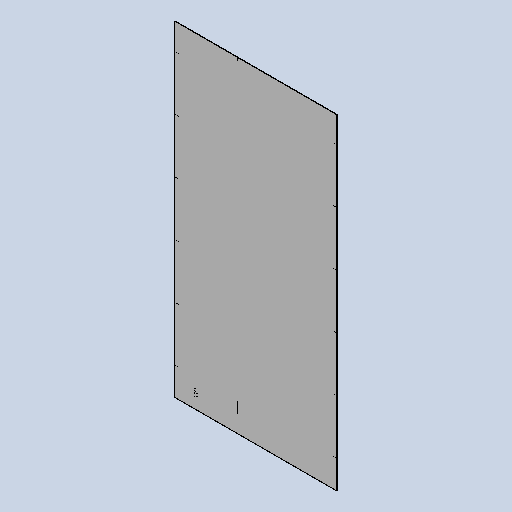
# Autodesk Inventor part: GBK 3122 shield 2
Saved by Autodesk Inventor 2026.2 (Build 302298010, 298A)
## iProperties
Created: 2026-04-17
Part Number: GBK 3122 shield 2
Material: Steel
Document SubType Name: Sheet Metal
Designer: pokla
Stock Number: 3122
Mass: 138487 g
Surface Area: 88564.8 cm^2
Volume: 17641.6 cm^3
Density: 7.85 g/cm^3
Flat Pattern Width: 298 cm
Flat Pattern Length: 148 cm
Flat Pattern Area: 44104 cm^2
Sheet Metal Rule: Default_mm
Sheet Metal Width: 2980,000 мм
Sheet Metal Length: 1480,000 мм
Sheet Metal Area: 4410400,000 мм^2
Appearance: Default
Author: admin
Autodesk Inventor part; units mm, degrees
ref_plane "YZ Plane" through (0, 0, 0) normal (1, 0, 0) x (0, 1, 0)
ref_plane "XZ Plane" through (0, 0, 0) normal (0, 1, 0) x (-1, 0, 0)
ref_plane "XY Plane" through (0, 0, 0) normal (0, 0, 1) x (1, 0, 0)
sketch "Sketch1" plane through (0, 0, 0) normal (0, 0, 1) x (1, 0, 0)
  line L0 (740, -1490) -> (-740, -1490)
  line L1 (-740, -1490) -> (-740, 1490)
  line L2 (-740, 1490) -> (740, 1490)
  line L3 (740, 1490) -> (740, -1490)
  line L4 (740, -1490) -> (-740, 1490) construction
  line L5 (-740, -1490) -> (740, 1490) construction
  point P0 (0, 0)
  dimension "d0" = 1480
  dimension "d1" = 2980
  measures "d0" distance of L1.end L2.end
  measures "d1" distance of L0.end L1.end
extrude "Plate1" add sketch "Sketch1" along normal blind 4
sketch "Эскиз5" plane through (0, 0, 0) normal (0, 0, -1) x (-1, 0, 0)
  line L0 (568.231, -1317.5249) -> (568.231, -1815.661) construction
  line L1 (568.231, -1815.661) -> (528.6037, -1815.661) construction
  line L2 (528.6037, -1815.661) -> (528.6037, -1317.5249) construction
  line L3 (528.6037, -1317.5249) -> (568.231, -1317.5249) construction
  line L4 (669.2463, -1238) -> (669.2463, -1335) projected
  line L5 (669.2463, -1335) -> (665.2463, -1335) projected
  line L6 (169.3732, -1238) -> (169.3732, -1335) projected
  line L7 (169.3732, -1335) -> (165.3732, -1335) projected
  line L8 (-330.5, -1238) -> (-330.5, -1335) projected
  line L9 (-330.5, -1335) -> (-334.5, -1335) projected
  line L10 (669.2463, 1460.5) -> (669.2463, 1520.5) projected
  line L11 (669.2463, 1460.5) -> (665.2463, 1460.5) projected
  line L12 (169.3732, 1460.5) -> (169.3732, 1520.5) projected
  line L13 (169.3732, 1460.5) -> (165.3732, 1460.5) projected
  line L14 (-330.5, 1460.5) -> (-330.5, 1520.5) projected
  line L15 (-330.5, 1460.5) -> (-334.5, 1460.5) projected
  line L16 (709.6246, -1234.5) -> (769.6246, -1234.5) projected
  line L17 (709.6246, -1234.5) -> (709.6246, -1230.5) projected
  line L18 (709.6246, -737.8333) -> (769.6246, -737.8333) projected
  line L19 (709.6246, -737.8333) -> (709.6246, -733.8333) projected
  line L20 (709.6246, -241.1667) -> (769.6246, -241.1667) projected
  line L21 (709.6246, -241.1667) -> (709.6246, -237.1667) projected
  line L22 (709.6246, 255.5) -> (769.6246, 255.5) projected
  line L23 (709.6246, 255.5) -> (709.6246, 259.5) projected
  line L24 (709.6246, 752.1667) -> (769.6246, 752.1667) projected
  line L25 (709.6246, 752.1667) -> (709.6246, 756.1667) projected
  line L26 (709.6246, 1248.8333) -> (769.6246, 1248.8333) projected
  line L27 (709.6246, 1248.8333) -> (709.6246, 1252.8333) projected
  line L28 (-740, -1234.5) -> (-710, -1234.5) projected
  line L29 (-710, -1234.5) -> (-710, -1230.5) projected
  line L30 (-740, -737.8333) -> (-710, -737.8333) projected
  line L31 (-710, -737.8333) -> (-710, -733.8333) projected
  line L32 (-740, -241.1667) -> (-710, -241.1667) projected
  line L33 (-710, -241.1667) -> (-710, -237.1667) projected
  line L34 (-740, 255.5) -> (-710, 255.5) projected
  line L35 (-710, 255.5) -> (-710, 259.5) projected
  line L36 (-740, 752.1667) -> (-710, 752.1667) projected
  line L37 (-710, 752.1667) -> (-710, 756.1667) projected
  line L38 (-740, 1248.8333) -> (-710, 1248.8333) projected
  line L39 (-710, 1248.8333) -> (-710, 1252.8333) projected
  point P0 (0, 0)
  constraints: 2 other
mark "Маркировка4"
equation "\"d0\" = Лист_ширина"
equation "\"d2\" = Thickness"
equation "\"BendRadius\" = Thickness"
equation "\"BendReliefWidth\" = Thickness"
equation "\"BendReliefDepth\" = 0.5 * Thickness"
equation "\"CornerReliefSize\" = 4 * Thickness"
equation "\"MinimumRemnant\" = 2 * Thickness"
equation "\"TransitionRadius\" = BendRadius"
equation "\"JacobiRadiusSize\" = BendRadius"
equation "\"GapSize\" = Thickness"
equation "\"Лист_ширина\" = 1480"
equation "\"Thickness\" = 4"
body "Solid1"
